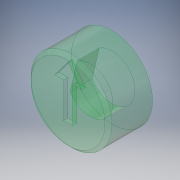
# Autodesk Inventor part: testpotcap
Saved by Autodesk Inventor 2017 SP1 (Build 210196100, 196)
## iProperties
Created: 2016-12-24
Part Number: testpotcap
Material: Generic
Document SubType Name: Modeling
Designer: wsh32
Density: 1 g/cm^3
Appearance: Clear - Green 1
Author: wsh32
Autodesk Inventor part; units mm, degrees
ref_plane "YZ Plane" through (0, 0, 0) normal (1, 0, 0) x (0, 1, 0)
ref_plane "XZ Plane" through (0, 0, 0) normal (0, 1, 0) x (-1, 0, 0)
ref_plane "XY Plane" through (0, 0, 0) normal (0, 0, 1) x (1, 0, 0)
sketch "Sketch1" plane through (0, 0, 0) normal (0, 0, 1) x (1, 0, 0)
  circle A0 centre (0, 0) radius 2.9845
  circle A1 centre (0, 0) radius 5.842
  circle A2 centre (0, 0) radius 3.302
  dimension "d0" = 5.969
  dimension "d2" = 0.3175
  dimension "d5" = 2.54
  constraints: 3 centre point, 1 coincident
  measures "d0" diameter of A0
  measures "d2" radial gap between concentric circles of A0 A2
  measures "d5" radial gap between concentric circles of A1 A2
extrude "Extrusion1" add sketch "Sketch1" along normal blind 25.4 contours A1
sketch "Sketch2" plane through (0, 0, 25.4) normal (0, 0, 1) x (1, 0, 0)
  circle A0 centre (0, 0) radius 5.842 projected
extrude "Extrusion2" add sketch "Sketch2" along normal blind 3.175
sketch "Sketch3" plane through (0, 0, 28.575) normal (0, 0, 1) x (1, 0, 0)
  line L0 (0.635, -2.54) -> (-0.635, -2.54)
  line L1 (-0.635, -2.54) -> (-0.635, 2.54)
  line L2 (-0.635, 2.54) -> (0.635, 2.54)
  line L3 (0.635, 2.54) -> (0.635, -2.54)
  line L4 (0.635, -2.54) -> (-0.635, 2.54) construction
  line L5 (-0.635, -2.54) -> (0.635, 2.54) construction
  line L6 (0, 2.54) -> (0, -2.54) construction
  line L7 (-1.905, 2.54) -> (1.905, 2.54)
  line L8 (1.905, 2.54) -> (0, 5.08)
  line L9 (0, 5.08) -> (-1.905, 2.54)
  point P0 (0, 0)
  dimension "d8" = 5.08
  dimension "d9" = 2.54
  dimension "d10" = 1.27
  dimension "d11" = 3.81
  constraints: 20 end point, 4 midpoint, 2 horizontal, 2 parallel, 1 collinear, 1 perpendicular, 1 point on line, 1 symmetric about line
  measures "d8" distance of L2.end L0.start
  measures "d9" distance from line of L8.end L7
  measures "d10" distance of L1.end L2.end
  measures "d11" distance of L7.start L7.end
extrude "Extrusion3" cut sketch "Sketch3" against normal blind 0.635
sketch "Sketch4" plane through (0, 0, 25.4) normal (0, 0, -1) x (-1, 0, 0)
  line L0 (0.635, -2.54) -> (0.635, 2.54) construction
  line L1 (0.635, 2.54) -> (1.905, 2.54) construction
  line L2 (1.905, 2.54) -> (0, 5.08) construction
  line L3 (0, 5.08) -> (-1.905, 2.54) construction
  line L4 (-1.905, 2.54) -> (-0.635, 2.54) construction
  line L5 (-0.635, 2.54) -> (-0.635, -2.54) construction
  line L6 (-0.635, -2.54) -> (0.635, -2.54) construction
  circle A0 centre (0, 0) radius 5.842 construction
  circle A1 centre (0, 0) radius 3.302 projected
  line L7 (1.8418, 2.7406) -> (2.8596, -1.651)
  line L8 (3.302, 0) -> (-3.302, 0) construction
  line L9 (-3.2774, -0.484) -> (-2.2595, -4.8756) construction
  line L10 (2.8596, 1.651) -> (1.8418, -2.7406) construction
  line L11 (-2.3742, 4.3806) -> (-3.3921, -0.011) construction
  line L12 (0, 0) -> (2.8596, 1.651) construction
  line L13 (0, 0) -> (2.8596, -1.651) construction
  dimension "d14" = 60
  dimension "d15" = 5.715
  constraints: 14 end point, 6 point on circle, 3 equal length, 2 parallel, 2 tangent, 1 horizontal, 1 midpoint, 1 symmetric about line
  measures "d14" angle of L13 L12
  measures "d15" distance between parallel lines of L9 L7
extrude "Extrusion4" add sketch "Sketch4" along normal blind 10.16 contours A1 L7 picked at (2.635, 0.6299)
sketch "Sketch5" plane through (0, 0, 28.575) normal (0, 0, 1) x (1, 0, 0)
  line L0 (-0.635, -2.54) -> (-0.635, 2.54) projected
  line L1 (-0.635, 2.54) -> (-1.905, 2.54) projected
  line L2 (-1.905, 2.54) -> (0, 5.08) projected
  line L3 (0, 5.08) -> (1.905, 2.54) projected
  line L4 (1.905, 2.54) -> (0.635, 2.54) projected
  line L5 (0.635, 2.54) -> (0.635, -2.54) projected
  line L6 (0.635, -2.54) -> (-0.635, -2.54) projected
  circle A0 centre (0, 0) radius 5.842 projected
extrude "Extrusion5" cut sketch "Sketch5" against normal blind 6.35 contours L0 L1 L2 L3 L4 L5 L6 | A0 keep common part
chamfer "Chamfer1" distance 0.508 angle 45 1 edges at (-5.842, 0, 28.575)
equation "\"d9\" = 0.5 * d8"
equation "\"d11\" = 3 * d10"
body "Solid1"
